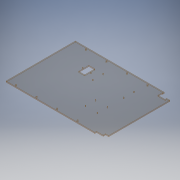
# Autodesk Inventor part: Acrylic_Panel_Mounts
Saved by Autodesk Inventor 2019.4 (Build 234330000, 330)
## iProperties
Created: 2020-01-31
Part Number: Acrylic_Panel_Mounts
Material: Generic
Document SubType Name: Modeling
Designer: Jorian Bruslind
Density: 1 g/cm^3
Appearance: Polycarbonate - Smoked
Author: Jorian Bruslind
Autodesk Inventor part; units mm, degrees
ref_plane "YZ Plane" through (0, 0, 0) normal (1, 0, 0) x (0, 1, 0)
ref_plane "XZ Plane" through (0, 0, 0) normal (0, 1, 0) x (-1, 0, 0)
ref_plane "XY Plane" through (0, 0, 0) normal (0, 0, 1) x (1, 0, 0)
sketch "Sketch1" plane through (0, 0, 0) normal (0, 1, 0) x (-1, 0, 0)
  line L0 (-240, 168.915) -> (240, 168.915)
  line L1 (240, 168.915) -> (240, -168.915)
  line L2 (240, -168.915) -> (-240, -168.915)
  line L3 (-240, -168.915) -> (-240, 168.915)
  line L4 (-240, 168.915) -> (240, -168.915) construction
  line L5 (240, 168.915) -> (-240, -168.915) construction
  point P0 (0, 0)
  dimension "d0" = 480
  dimension "d1" = 337.83
  constraints: 12 end point, 2 midpoint, 2 parallel, 1 horizontal, 1 perpendicular
  measures "d0" distance of L1.end L2.end
  measures "d1" distance of L0.end L1.end
extrude "Extrusion1" add sketch "Sketch1" along normal blind 5
sketch "Sketch2" plane through (0, 5, 0) normal (0, 1, 0) x (1, 0, 0)
  line L0 (240, -168.915) -> (240, 168.915) projected
  line L1 (240, -168.915) -> (240, -148.915)
  line L2 (240, -148.915) -> (225, -148.915)
  line L3 (-240, -168.915) -> (240, -168.915) projected
  line L4 (225, -168.915) -> (225, -160.915)
  line L5 (225, -168.915) -> (233, -168.915) construction
  line L6 (225, -148.915) -> (225, -160.915)
  line L7 (225, -160.915) -> (193, -160.915)
  line L8 (193, -160.915) -> (193, -168.915)
  line L9 (193, -168.915) -> (240, -168.915)
  line L10 (240, 0) -> (160.3142, 0)
  line L11 (240, 168.915) -> (240, 148.915)
  line L12 (240, 148.915) -> (225, 148.915)
  line L13 (225, 168.915) -> (225, 160.915)
  line L14 (225, 168.915) -> (233, 168.915) construction
  line L15 (225, 148.915) -> (225, 160.915)
  line L16 (225, 160.915) -> (193, 160.915)
  line L17 (193, 160.915) -> (193, 168.915)
  line L18 (193, 168.915) -> (240, 168.915)
  point P0 (0, 0)
  dimension "d4" = 20
  dimension "d5" = 15
  dimension "d6" = 8
  dimension "d7" = 90
  dimension "d8" = 12
  dimension "d9" = 32
  constraints: 34 end point, 7 symmetric about line, 5 perpendicular, 3 horizontal, 3 point on line, 1 midpoint, 1 vertical
  measures "d4" distance of L0.start L1.end
  measures "d5" distance of L1.end L2.end
  measures "d6" distance of L4.start L4.end
  measures "d7" angle of L5 L4
  measures "d8" distance of L2.end L4.end
  measures "d9" distance of L4.end L7.end
extrude "Extrusion2" cut sketch "Sketch2" against normal blind 5
sketch "Sketch4" plane through (0, 5, 0) normal (0, 1, 0) x (1, 0, 0)
  line L0 (-240, -168.915) -> (193, -168.915) projected
  line L1 (-240, -168.915) -> (-200, -168.915)
  line L2 (-200, -168.915) -> (-200, -160.183)
  circle A0 centre (-200, -160.183) radius 2.75
  circle A1 centre (-100, -160.183) radius 2.75
  circle A2 centre (0, -160.183) radius 2.75
  circle A3 centre (100, -160.183) radius 2.75
  line L3 (193, 168.915) -> (-240, 168.915) projected
  line L4 (-240, 168.915) -> (-180, 168.915)
  line L5 (-180, 168.915) -> (-180, 160.183)
  circle A4 centre (-180, 160.183) radius 2.75
  circle A5 centre (-80, 160.183) radius 2.75
  circle A6 centre (20, 160.183) radius 2.75
  circle A7 centre (120, 160.183) radius 2.75
  point P0 (0, 0)
  dimension "d14" = 40
  dimension "d15" = 8.732
  dimension "d16" = 5.5
  dimension "d19" = 100
  dimension "d24" = 60
  dimension "d25" = 8.732
  dimension "d26" = 5.5
  dimension "d29" = 100
  constraints: 8 centre point, 8 end point, 2 coincident, 2 horizontal, 2 perpendicular, 2 point on line, 12 other
  measures "d14" distance of L0.start L1.end
  measures "d15" distance of L1.end L2.end
  measures "d16" diameter of A0
  measures "d19" distance of A0.centre A1.centre
  measures "d24" distance of L3.end L4.end
  measures "d25" distance of L4.end L5.end
  measures "d26" diameter of A4
  measures "d29" distance of A4.centre A5.centre
extrude "Extrusion3" cut sketch "Sketch4" against normal blind 10
sketch "Sketch5" plane through (0, 5, 0) normal (0, 1, 0) x (1, 0, 0)
  line L0 (193, 168.915) -> (-240, 168.915) projected
  line L1 (-240, 168.915) -> (240, 168.915)
  line L2 (240, 168.915) -> (240, -170.085)
  line L3 (240, -170.085) -> (-240, -170.085)
  line L4 (-240, -170.085) -> (-240, 168.915)
  point P0 (0, 0)
  dimension "d36" = 480
  dimension "d37" = 339
  constraints: 8 end point, 2 parallel, 1 horizontal, 1 perpendicular
  measures "d36" distance of L2.end L3.end
  measures "d37" distance of L1.end L2.end
sketch "Sketch8" plane through (0, 5, 0) normal (0, 1, 0) x (1, 0, 0)
  line L0 (193, 160.915) -> (225, 160.915) projected
  line L1 (225, 160.915) -> (190, 160.915)
  line L2 (190, 160.915) -> (190, 140.915)
  line L3 (190, 140.915) -> (225, 140.915)
  line L4 (225, 140.915) -> (225, 160.915)
  point P0 (0, 0)
  dimension "d38" = 35
  dimension "d39" = 20
  constraints: 8 end point, 2 parallel, 1 horizontal, 1 perpendicular
  measures "d38" distance of L3.end L2.end
  measures "d39" distance of L2.end L1.end
extrude "Extrusion4" cut sketch "Sketch8" against normal blind 10
sketch "Sketch9" plane through (0, 5, 0) normal (0, 1, 0) x (1, 0, 0)
  circle A0 centre (115, 98.915) radius 2
  line L0 (193, 168.915) -> (-240, 168.915) projected
  line L1 (240, -148.915) -> (240, 148.915) projected
  circle A1 centre (115, 48.915) radius 2
  circle A2 centre (-35, 98.915) radius 2
  circle A3 centre (-35, 48.915) radius 2
  line L2 (-35, 98.915) -> (-75, 98.915)
  line L3 (-35, 98.915) -> (5, 98.915) construction
  line L4 (-75, 98.915) -> (-75, 83.915)
  line L5 (-75, 83.915) -> (-75, 98.915)
  line L6 (-75, 98.915) -> (-104, 98.915)
  line L7 (-104, 98.915) -> (-104, 48.915)
  line L8 (-104, 48.915) -> (-75, 48.915)
  line L9 (-75, 48.915) -> (-75, 98.915)
  line L10 (-104, 73.915) -> (-109.5, 73.915)
  line L11 (-75, 73.915) -> (-69.5, 73.915)
  circle A4 centre (-69.5, 73.915) radius 1.75
  circle A5 centre (-109.5, 73.915) radius 1.75
  circle A6 centre (115, -78.915) radius 1.75
  line L12 (-240, -168.915) -> (193, -168.915) projected
  circle A7 centre (57, -78.915) radius 1.75
  circle A8 centre (115, -29.915) radius 1.75
  circle A9 centre (57, -29.915) radius 1.75
  point P0 (0, 0)
  dimension "d42" = 4
  dimension "d43" = 70
  dimension "d44" = 125
  dimension "d47" = 50
  dimension "d50" = 150
  dimension "d53" = 40
  dimension "d54" = 180
  dimension "d55" = 15
  dimension "d56" = 15
  dimension "d57" = 29
  dimension "d58" = 50
  dimension "d59" = 5.5
  dimension "d60" = 5.5
  dimension "d61" = 3.5
  dimension "d62" = 3.5
  dimension "d63" = 3.5
  dimension "d64" = 90
  dimension "d65" = 125
  dimension "d68" = 58
  dimension "d71" = 49
  constraints: 20 end point, 10 centre point, 7 horizontal, 3 vertical, 2 coincident, 2 midpoint, 2 parallel, 1 collinear, 1 perpendicular, 1 point on line, 12 other
  measures "d42" diameter of A0
  measures "d43" distance from line of L0 A0.centre
  measures "d44" distance from line of L1 A0.centre
  measures "d47" distance of A0.centre A1.centre
  measures "d50" distance of A0.centre L2.start
  measures "d53" distance of L2.start L2.end
  measures "d54" angle of L2 L3
  measures "d55" distance of L2.end L4.end
  measures "d56" distance of L4.end L5.end
  measures "d57" distance of L8.end L7.end
  measures "d58" distance of L7.end L6.end
  measures "d59" distance of L10.start L10.end
  measures "d60" distance of L11.start L11.end
  measures "d61" diameter of A4
  measures "d62" diameter of A5
  measures "d63" diameter of A6
  measures "d64" distance from line of L12 A6.centre
  measures "d65" distance from line of L1 A6.centre
  measures "d68" distance of A6.centre A7.centre
  measures "d71" distance of A6.centre A8.centre
extrude "Extrusion5" cut sketch "Sketch9" against normal blind 10
body "Solid1"
